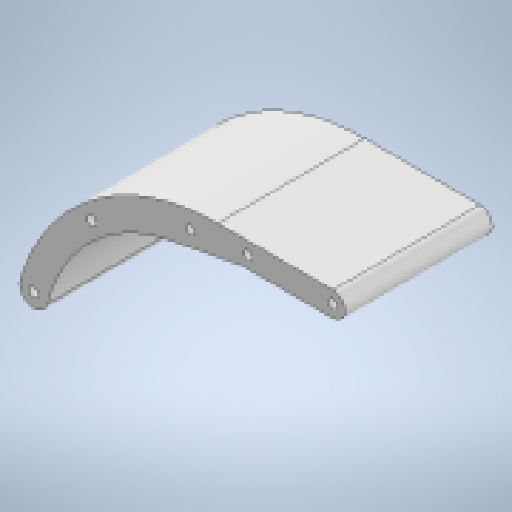
# Autodesk Inventor part: tesaki_sukima
Saved by Autodesk Inventor 2025.1 (Build 291241000, 241)
## iProperties
Created: 2024-09-04
Part Number: tesaki_sukima
Material: ABS プラスチック
Document SubType Name: Modeling
Designer: right
Mass: 8.72097 g
Surface Area: 49.8477 cm^2
Volume: 8.22733 cm^3
Density: 1.06 g/cm^3
Appearance: 滑らか - 白
Author: right
Autodesk Inventor part; units mm, degrees
ref_plane "YZ Plane" through (0, 0, 0) normal (1, 0, 0) x (0, 1, 0)
ref_plane "XZ Plane" through (0, 0, 0) normal (0, 1, 0) x (-1, 0, 0)
sketch "スケッチ1" plane through (0, 0, 0) normal (0, 0, 1) x (1, 0, 0)
  circle A0 centre (-4.6538, 21.3462) radius 1.1 projected
  circle A1 centre (-19.6538, 21.3462) radius 1.1 projected
  line L0 (0.5, 16.7574) -> (0.5, 6.421) projected
  arc A2 (-3.1924, 5.3553) -> (0.5, 6.421) centre (-1.5, 6.421) ccw projected
  arc A3 (-3.1924, 5.3553) -> (-13.8372, 15.4455) centre (-28.2569, -10.4267) ccw projected
  arc A4 (-12.8636, 19.1925) -> (-13.8372, 15.4455) centre (-12.8636, 17.1925) ccw projected
  line L1 (-12.8636, 19.1925) -> (-2.3985, 19.1925) projected
  arc A5 (-1.3325, 18.8847) -> (-2.3985, 19.1925) centre (-2.3985, 17.1925) ccw projected
  arc A6 (-1.3325, 18.8847) -> (-0.8333, 18.643) centre (0, 21) ccw projected
  arc A7 (0.5, 16.7574) -> (-0.8333, 18.643) centre (-1.5, 16.7574) ccw projected
  arc A8 (-2.3454, -0.8655) -> (2.5, 0) centre (0, 0) ccw projected
  line L2 (2.5, 0) -> (2.5, 16.5) projected
  arc A9 (4.5, 18.5) -> (2.5, 16.5) centre (4.5, 16.5) ccw projected
  line L3 (4.5, 18.5) -> (21, 18.5) projected
  arc A10 (21, 18.5) -> (21, 23.5) centre (21, 21) ccw projected
  line L4 (21, 23.5) -> (-25, 23.5) projected
  arc A11 (-25, 23.5) -> (-59.8955, -2.5) centre (-25, -12.9173) ccw projected
  arc A12 (-59.8955, -2.5) -> (-55.0727, -3.8137) centre (-57.5, -3.2151) ccw projected
  arc A13 (-2.3454, -0.8655) -> (-55.0727, -3.8137) centre (-28.2569, -10.4267) ccw projected
  circle A14 centre (0, 0) radius 1.1 projected
  circle A15 centre (-47.2894, 12.7841) radius 1.1 projected
  circle A16 centre (-29.7988, 20.1536) radius 1.1 projected
  circle A17 centre (0, 21) radius 1.1 projected
  circle A18 centre (-57.5, -3.2151) radius 1.1 projected
  circle A19 centre (21, 21) radius 1.1 projected
  line L5 (-12.8636, 19.1925) -> (-20.8636, 19.1925)
  line L6 (-33.6212, 16.6665) -> (-20.8636, 19.1925)
  circle A20 centre (-57.5, -3.2151) radius 0.8
  circle A21 centre (-47.2894, 12.7841) radius 0.8
  circle A22 centre (-29.7988, 20.1536) radius 0.8
  circle A23 centre (-19.6538, 21.3462) radius 0.8
  circle A24 centre (-4.6538, 21.3462) radius 0.8
  circle A25 centre (-4.6538, 21.3462) radius 2.1538
  point P0 (0, 0)
  point P1 (-4.6538, 19.1925)
  point P2 (-4.6538, 23.5)
  dimension "d0" = 8
  dimension "d1" = 1.6
  dimension "d2" = 1.6
  dimension "d3" = 1.6
  dimension "d4" = 1.6
  dimension "d5" = 1.6
  constraints: 6 centre point, 6 coincident, 4 end point, 2 tangent, 1 horizontal, 1 point on circle
  measures "d0" distance of L1.start L5.end
  measures "d1" diameter of A20
  measures "d2" diameter of A21
  measures "d3" diameter of A22
  measures "d4" diameter of A23
  measures "d5" diameter of A24
ref_plane "作業平面1" through (-60, -5.7151, 26) normal (0, 0, -1) x (0, 1, 0)
extrude "押し出し1" add sketch "スケッチ1" along normal up to surface (26 mm away) contours A0 | A1 | L5 L6 A13 A12 A11 L4 A25 L1 | A25 | A15 | A16 | A18
fillet "フィレット1" radius 2 1 edges at (-20.8636, 19.1925, 13)
